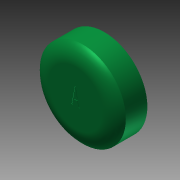
# Autodesk Inventor part: A Button
Saved by Autodesk Inventor 2012 SP1 (Build 160190100, 190)
## iProperties
Created: 2011-12-05
Part Number: A Button
Material: Default
Document SubType Name: Modeling
Designer: 133098
Density: 1 g/cm^3
Author: 133098
Autodesk Inventor part; units mm, degrees
ref_plane "YZ Plane" through (0, 0, 0) normal (1, 0, 0) x (0, 1, 0)
ref_plane "XZ Plane" through (0, 0, 0) normal (0, 1, 0) x (-1, 0, 0)
ref_plane "XY Plane" through (0, 0, 0) normal (0, 0, 1) x (1, 0, 0)
sketch "Sketch1" plane through (0, 0, 0) normal (0, 0, 1) x (1, 0, 0)
  circle A0 centre (0, 0) radius 7.62
  dimension "d0" = 15.24
  constraints: 1 centre point, 1 coincident
  measures "d0" diameter of A0
extrude "Extrusion1" add sketch "Sketch1" along normal blind 5.08
chamfer "Chamfer1" distance 1.27 angle 45 1 edges at (-7.62, 0, 5.08)
fillet "Fillet1" radius 3.81 1 edges at (-6.35, 0, 5.08)
sketch "Sketch2" plane through (0, 0, 5.08) normal (0, 0, 1) x (1, 0, 0)
  line L0 (-0.7017, 1.8442) -> (0.7248, 1.8442) construction
  line L1 (0.7248, 1.8442) -> (0.7248, -1.2038) construction
  line L2 (0.7248, -1.2038) -> (-0.7017, -1.2038) construction
  line L3 (-0.7017, -1.2038) -> (-0.7017, 1.8442) construction
  line L4 (-0.704, -1.2038) -> (-0.1186, 1.8442)
  line L5 (-0.1186, 1.8442) -> (0.0975, 1.8442)
  line L6 (0.0975, 1.8442) -> (0.7224, -1.2038)
  line L7 (0.7224, -1.2038) -> (0.4924, -1.2038)
  line L8 (0.4924, -1.2038) -> (0.3159, -0.2815)
  line L9 (0.3159, -0.2815) -> (-0.3253, -0.2815)
  line L10 (-0.3253, -0.2815) -> (-0.4903, -1.2038)
  line L11 (-0.4903, -1.2038) -> (-0.704, -1.2038)
  line L12 (-0.2649, 0.0461) -> (0.2531, 0.0461)
  line L13 (0.2531, 0.0461) -> (0.0952, 0.8917)
  spline S0 degree 2 poles (0.0952, 0.8917) (0.0208, 1.2774) (-0.014, 1.5236) knots 0 0 0 1 1 1
  spline S1 degree 2 poles (-0.014, 1.5236) (-0.0442, 1.2309) (-0.0976, 0.9428) knots 0 0 0 1 1 1
  line L14 (-0.0976, 0.9428) -> (-0.2649, 0.0461)
  constraints: 2 other
extrude "Extrusion2" cut sketch "Sketch2" against normal blind 0.0635
body "Solid1"
